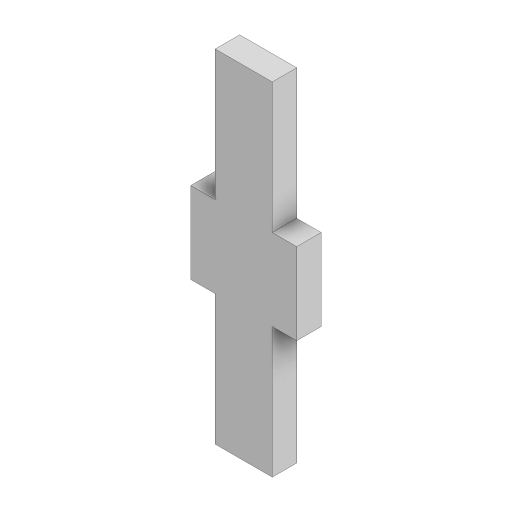
# Autodesk Inventor part: Side piece 2 2x
Saved by Autodesk Inventor 2023.3 (Build 273359000, 359)
## iProperties
Created: 2024-09-20
Part Number: Side piece 2 2x
Material: Generic
Document SubType Name: Modeling
Designer: David Zindović
Density: 1 g/cm^3
Appearance: Default
Author: David Zindović
Autodesk Inventor part; units mm, degrees
ref_plane "YZ Plane" through (0, 0, 0) normal (1, 0, 0) x (0, 1, 0)
ref_plane "XZ Plane" through (0, 0, 0) normal (0, 1, 0) x (-1, 0, 0)
ref_plane "XY Plane" through (0, 0, 0) normal (0, 0, 1) x (1, 0, 0)
sketch "Sketch1" plane through (0, 0, 0) normal (0, 0, 1) x (1, 0, 0)
  line L0 (-6.5, 24) -> (6.5, 24)
  line L1 (6.5, 24) -> (6.5, -24)
  line L2 (6.5, -24) -> (-6.5, -24)
  line L3 (-6.5, -24) -> (-6.5, 24)
  line L4 (-6.5, 5) -> (-3.5, 5)
  line L5 (-3.5, 5) -> (-3.5, -5)
  line L6 (-3.5, -5) -> (-6.5, -5)
  line L7 (-6.5, -5) -> (-6.5, 5)
  line L8 (-3.5, 24) -> (3.5, 24)
  line L9 (3.5, 24) -> (3.5, 21)
  line L10 (3.5, 21) -> (-3.5, 21)
  line L11 (-3.5, 21) -> (-3.5, 24)
  line L12 (0, 0) -> (0.5, 0)
  line L13 (0, 0) -> (0, -2.6489)
  line L14 (6.5, 5) -> (3.5, 5)
  line L15 (3.5, 5) -> (3.5, -5)
  line L16 (3.5, -5) -> (6.5, -5)
  line L17 (3.5, -24) -> (3.5, -21)
  line L18 (3.5, -21) -> (-3.5, -21)
  line L19 (-3.5, -21) -> (-3.5, -24)
  line L20 (-3.5, -5) -> (-3.5, -24)
  line L21 (-3.5, 5) -> (-3.5, 24)
  line L22 (3.5, 24) -> (3.5, 5)
  line L23 (3.5, -5) -> (3.5, -24)
  point P0 (0, 24)
  point P1 (6.5, 0)
  point P2 (-3.5, 0)
  point P3 (0, 21)
  point P4 (0, -21)
  point P5 (6.5, 5)
  point P6 (6.5, -5)
  point P7 (3.5, 21)
  point P8 (3.5, -21)
  point P9 (3.5, 21)
  point P10 (-3.5, 21)
  point P11 (-3.5, -21)
  point P12 (3.5, -21)
  dimension "d0" = 48
  dimension "d1" = 13
  dimension "d2" = 3
  dimension "d3" = 10
  dimension "d4" = 7
  dimension "d5" = 3
  constraints: 46 end point, 9 symmetric about line, 6 parallel, 4 horizontal, 4 midpoint, 3 perpendicular, 2 horizontal alignment, 2 point on line, 2 vertical alignment, 1 vertical, 3 other
  measures "d0" distance of L0.end L1.end
  measures "d1" distance of L0.start L0.end
  measures "d2" distance of L5.end L6.end
  measures "d3" distance of L4.end L5.end
  measures "d4" distance of L9.end L10.end
  measures "d5" distance of L8.end L9.end
extrude "Extrusion1" add sketch "Sketch1" along normal mid plane 3 contours L4 L5 L6 L3 | L10 L22 L15 L23 L18 L20 L5 L21 | L1 L16 L15 L14
body "Solid1"
